Autodesk Fusion 360 part; units mm, degrees
(part 2 of 2)
sketch "Sketch26" plane through (0, 0, 45.5) normal (0, 0, 1) x (-1, 0, 0)
  line L0 (180, -249) -> (180, -94.7885)
  line L1 (180, -94.7885) -> (6, -94.7885)
  line L2 (6, -94.7885) -> (6, -109.4985)
  line L3 (6, -109.4985) -> (-58, -109.4985)
  line L4 (-58, -109.4985) -> (-58, -249)
  line L5 (-58, -249) -> (180, -249)
  circle A0 centre (58, -179.8487) radius 2.75
  circle A1 centre (58, -204.6724) radius 2.75
  circle A2 centre (58, -154.7263) radius 2.75
  circle A3 centre (58, -230.0227) radius 2.75
  circle A4 centre (58, -129.8013) radius 2.75
  line L6 (170, -234) -> (70, -234)
  line L7 (70, -229) -> (170, -229)
  arc A5 (170, -234) -> (170, -229) centre (170, -231.5) ccw
  arc A6 (70, -229) -> (70, -234) centre (70, -231.5) ccw
  line L8 (70, -219.3846) -> (170, -219.3846)
  line L9 (170, -224.3846) -> (70, -224.3846)
  arc A7 (170, -224.3846) -> (170, -219.3846) centre (170, -221.8846) ccw
  arc A8 (70, -219.3846) -> (70, -224.3846) centre (70, -221.8846) ccw
  line L10 (70, -209.7692) -> (170, -209.7692)
  line L11 (170, -214.7692) -> (70, -214.7692)
  arc A9 (170, -214.7692) -> (170, -209.7692) centre (170, -212.2692) ccw
  arc A10 (70, -209.7692) -> (70, -214.7692) centre (70, -212.2692) ccw
  line L12 (70, -200.1538) -> (170, -200.1538)
  line L13 (170, -205.1538) -> (70, -205.1538)
  arc A11 (170, -205.1538) -> (170, -200.1538) centre (170, -202.6538) ccw
  arc A12 (70, -200.1538) -> (70, -205.1538) centre (70, -202.6538) ccw
  line L14 (70, -180.9231) -> (170, -180.9231)
  line L15 (170, -185.9231) -> (70, -185.9231)
  arc A13 (170, -185.9231) -> (170, -180.9231) centre (170, -183.4231) ccw
  arc A14 (70, -180.9231) -> (70, -185.9231) centre (70, -183.4231) ccw
  line L16 (70, -152.0769) -> (170, -152.0769)
  line L17 (170, -157.0769) -> (70, -157.0769)
  arc A15 (170, -157.0769) -> (170, -152.0769) centre (170, -154.5769) ccw
  arc A16 (70, -152.0769) -> (70, -157.0769) centre (70, -154.5769) ccw
  line L18 (70, -123.2308) -> (170, -123.2308)
  line L19 (170, -128.2308) -> (70, -128.2308)
  arc A17 (170, -128.2308) -> (170, -123.2308) centre (170, -125.7308) ccw
  arc A18 (70, -123.2308) -> (70, -128.2308) centre (70, -125.7308) ccw
  line L20 (70, -104) -> (170, -104)
  line L21 (170, -109) -> (70, -109)
  arc A19 (170, -109) -> (170, -104) centre (170, -106.5) ccw
  arc A20 (70, -104) -> (70, -109) centre (70, -106.5) ccw
  dimension "d193" = 5
  dimension "d194" = 5
  dimension "d197" = 0
  dimension "d198" = 125
  constraint horizontal L6
  constraint horizontal L7
  measures "d193" diameter of A6
  measures "d194" diameter of A5
extrude "Extrude39" cut sketch "Sketch26" against normal blind 15 contours L6 L7 A5 A6 | L8 L9 A7 A8 | L10 L11 A9 A10 | L12 L13 A11 A12 | L14 L15 A13 A14 | L16 L17 A15 A16 | L18 L19 A17 A18 | L20 L21 A19 A20 bodies 8
sketch "Sketch27" plane through (0, 69, 0) normal (0, 1, 0) x (-1, 0, 0)
  line L0 (-29.7143, 10) -> (-29.7143, 35)
  arc A0 (-24.7143, 35) -> (-29.7143, 35) centre (-27.2143, 35) ccw
  line L1 (-24.7143, 35) -> (-24.7143, 10)
  arc A1 (-29.7143, 10) -> (-24.7143, 10) centre (-27.2143, 10) ccw
  line L2 (8.8571, 10) -> (8.8571, 35)
  arc A2 (13.8571, 35) -> (8.8571, 35) centre (11.3571, 35) ccw
  line L3 (13.8571, 35) -> (13.8571, 10)
  arc A3 (8.8571, 10) -> (13.8571, 10) centre (11.3571, 10) ccw
  line L4 (66.7143, 10) -> (66.7143, 35)
  arc A4 (71.7143, 35) -> (66.7143, 35) centre (69.2143, 35) ccw
  line L5 (71.7143, 35) -> (71.7143, 10)
  arc A5 (66.7143, 10) -> (71.7143, 10) centre (69.2143, 10) ccw
  line L6 (76.3571, 10) -> (76.3571, 35)
  arc A6 (81.3571, 35) -> (76.3571, 35) centre (78.8571, 35) ccw
  line L7 (81.3571, 35) -> (81.3571, 10)
  arc A7 (76.3571, 10) -> (81.3571, 10) centre (78.8571, 10) ccw
  line L8 (18.5, 10) -> (18.5, 35)
  arc A8 (23.5, 35) -> (18.5, 35) centre (21, 35) ccw
  line L9 (23.5, 35) -> (23.5, 10)
  arc A9 (18.5, 10) -> (23.5, 10) centre (21, 10) ccw
  line L10 (-20.0714, 10) -> (-20.0714, 35)
  arc A10 (-15.0714, 35) -> (-20.0714, 35) centre (-17.5714, 35) ccw
  line L11 (-15.0714, 35) -> (-15.0714, 10)
  arc A11 (-20.0714, 10) -> (-15.0714, 10) centre (-17.5714, 10) ccw
  line L12 (-39.3571, 10) -> (-39.3571, 35)
  arc A12 (-34.3571, 35) -> (-39.3571, 35) centre (-36.8571, 35) ccw
  line L13 (-34.3571, 35) -> (-34.3571, 10)
  arc A13 (-39.3571, 10) -> (-34.3571, 10) centre (-36.8571, 10) ccw
  line L14 (-0.7857, 10) -> (-0.7857, 35)
  arc A14 (4.2143, 35) -> (-0.7857, 35) centre (1.7143, 35) ccw
  line L15 (4.2143, 35) -> (4.2143, 10)
  arc A15 (-0.7857, 10) -> (4.2143, 10) centre (1.7143, 10) ccw
  line L16 (57.0714, 10) -> (57.0714, 35)
  arc A16 (62.0714, 35) -> (57.0714, 35) centre (59.5714, 35) ccw
  line L17 (62.0714, 35) -> (62.0714, 10)
  arc A17 (57.0714, 10) -> (62.0714, 10) centre (59.5714, 10) ccw
  line L18 (86, 10) -> (86, 35)
  arc A18 (91, 35) -> (86, 35) centre (88.5, 35) ccw
  line L19 (91, 35) -> (91, 10)
  arc A19 (86, 10) -> (91, 10) centre (88.5, 10) ccw
  line L20 (47.4286, 10) -> (47.4286, 35)
  arc A20 (52.4286, 35) -> (47.4286, 35) centre (49.9286, 35) ccw
  line L21 (52.4286, 35) -> (52.4286, 10)
  arc A21 (47.4286, 10) -> (52.4286, 10) centre (49.9286, 10) ccw
  line L22 (-10.4286, 10) -> (-10.4286, 35)
  arc A22 (-5.4286, 35) -> (-10.4286, 35) centre (-7.9286, 35) ccw
  line L23 (-5.4286, 35) -> (-5.4286, 10)
  arc A23 (-10.4286, 10) -> (-5.4286, 10) centre (-7.9286, 10) ccw
  line L24 (-49, 10) -> (-49, 35)
  arc A24 (-44, 35) -> (-49, 35) centre (-46.5, 35) ccw
  line L25 (-44, 35) -> (-44, 10)
  arc A25 (-49, 10) -> (-44, 10) centre (-46.5, 10) ccw
  line L26 (180, 3) -> (-58, 3)
  line L27 (180, 3) -> (180, 61)
  line L28 (180, 61) -> (-58, 61)
  line L29 (-58, 61) -> (-58, 3)
  circle A26 centre (34, 14) radius 7
  line L30 (100, 35) -> (100, 10)
  line L31 (95, 10) -> (95, 35)
  arc A27 (100, 35) -> (95, 35) centre (97.5, 35) ccw
  arc A28 (95, 10) -> (100, 10) centre (97.5, 10) ccw
  line L32 (109.7143, 35) -> (109.7143, 10)
  line L33 (104.7143, 10) -> (104.7143, 35)
  arc A29 (109.7143, 35) -> (104.7143, 35) centre (107.2143, 35) ccw
  arc A30 (104.7143, 10) -> (109.7143, 10) centre (107.2143, 10) ccw
  line L34 (119.4286, 35) -> (119.4286, 10)
  line L35 (114.4286, 10) -> (114.4286, 35)
  arc A31 (119.4286, 35) -> (114.4286, 35) centre (116.9286, 35) ccw
  arc A32 (114.4286, 10) -> (119.4286, 10) centre (116.9286, 10) ccw
  line L36 (129.1429, 35) -> (129.1429, 10)
  line L37 (124.1429, 10) -> (124.1429, 35)
  arc A33 (129.1429, 35) -> (124.1429, 35) centre (126.6429, 35) ccw
  arc A34 (124.1429, 10) -> (129.1429, 10) centre (126.6429, 10) ccw
  line L38 (138.8571, 35) -> (138.8571, 10)
  line L39 (133.8571, 10) -> (133.8571, 35)
  arc A35 (138.8571, 35) -> (133.8571, 35) centre (136.3571, 35) ccw
  arc A36 (133.8571, 10) -> (138.8571, 10) centre (136.3571, 10) ccw
  line L40 (148.5714, 35) -> (148.5714, 10)
  line L41 (143.5714, 10) -> (143.5714, 35)
  arc A37 (148.5714, 35) -> (143.5714, 35) centre (146.0714, 35) ccw
  arc A38 (143.5714, 10) -> (148.5714, 10) centre (146.0714, 10) ccw
  line L42 (158.2857, 35) -> (158.2857, 10)
  line L43 (153.2857, 10) -> (153.2857, 35)
  arc A39 (158.2857, 35) -> (153.2857, 35) centre (155.7857, 35) ccw
  arc A40 (153.2857, 10) -> (158.2857, 10) centre (155.7857, 10) ccw
  line L44 (168, 35) -> (168, 10)
  line L45 (163, 10) -> (163, 35)
  arc A41 (168, 35) -> (163, 35) centre (165.5, 35) ccw
  arc A42 (163, 10) -> (168, 10) centre (165.5, 10) ccw
  dimension "d201" = 5
  dimension "d202" = 5
  dimension "d205" = 68
  dimension "d206" = 0
  constraint vertical L30
  constraint vertical L31
  measures "d201" diameter of A27
  measures "d202" diameter of A28
sketch "Sketch28" plane through (0, 69, 0) normal (0, 1, 0) x (-1, 0, 0)
extrude "Extrude40" cut sketch "Sketch27" against normal blind 10 contours L30 L31 A27 A28 | L32 L33 A29 A30 | L34 L35 A31 A32 | L36 L37 A33 A34 | L38 L39 A35 A36 | L40 L41 A37 A38 | L42 L43 A39 A40 | L44 L45 A41 A42 bodies 2
fillet "Fillet16" radius 2.5 20 edges at (-95, -75.9913, 57) (-103, -75.9913, 57) (-111, -75.9913, 57) (-119, -75.9913, 57) (-127, -75.9913, 57) (-135, -76, 57) (-143, -76, 57) (-151, -76, 57) (-159, -76, 57) (-167, -75.9913, 57) (-172, -75.9913, 57) (-164, -75.9913, 57) (-156, -76, 57) (-148, -76, 57) (-140, -76, 57) (-132, -75.9913, 57) (-124, -75.9913, 57) (-116, -75.9913, 57) (-108, -75.9913, 57) (-100, -75.9913, 57) on bodies 2
extrude "Extrude41" cut sketch "Sketch23" against normal blind 235 bodies 2
sketch "Sketch29" plane through (0, -79, 0) normal (0, -1, 0) x (1, 0, 0)
  line L0 (-95, 54.5) -> (-95, 10)
  arc A0 (-100, 10) -> (-95, 10) centre (-97.5, 10) ccw
  line L1 (-100, 10) -> (-100, 54.5)
  arc A1 (-97.5, 57) -> (-100, 54.5) centre (-97.5, 54.5) ccw
  arc A2 (-95, 54.5) -> (-97.5, 57) centre (-97.5, 54.5) ccw
  line L2 (-8.0005, 61) -> (-180, 61)
  line L3 (-180, 61) -> (-180, 3)
  line L4 (-8.0005, 3) -> (-180, 3)
  line L5 (-8.0005, 3) -> (-8.0005, 61)
  line L6 (-167, 54.5) -> (-167, 10)
  arc A3 (-172, 10) -> (-167, 10) centre (-169.5, 10) ccw
  line L7 (-172, 10) -> (-172, 54.5)
  arc A4 (-169.5, 57) -> (-172, 54.5) centre (-169.5, 54.5) ccw
  arc A5 (-167, 54.5) -> (-169.5, 57) centre (-169.5, 54.5) ccw
  line L8 (-159, 54.5) -> (-159, 10)
  arc A6 (-164, 10) -> (-159, 10) centre (-161.5, 10) ccw
  line L9 (-164, 10) -> (-164, 54.5)
  arc A7 (-161.5, 57) -> (-164, 54.5) centre (-161.5, 54.5) ccw
  arc A8 (-159, 54.5) -> (-161.5, 57) centre (-161.5, 54.5) ccw
  line L10 (-151, 54.5) -> (-151, 10)
  arc A9 (-156, 10) -> (-151, 10) centre (-153.5, 10) ccw
  line L11 (-156, 10) -> (-156, 54.5)
  arc A10 (-153.5, 57) -> (-156, 54.5) centre (-153.5, 54.5) ccw
  arc A11 (-151, 54.5) -> (-153.5, 57) centre (-153.5, 54.5) ccw
  line L12 (-143, 54.5) -> (-143, 10)
  arc A12 (-148, 10) -> (-143, 10) centre (-145.5, 10) ccw
  line L13 (-148, 10) -> (-148, 54.5)
  arc A13 (-145.5, 57) -> (-148, 54.5) centre (-145.5, 54.5) ccw
  arc A14 (-143, 54.5) -> (-145.5, 57) centre (-145.5, 54.5) ccw
  line L14 (-135, 54.5) -> (-135, 10)
  arc A15 (-140, 10) -> (-135, 10) centre (-137.5, 10) ccw
  line L15 (-140, 10) -> (-140, 54.5)
  arc A16 (-137.5, 57) -> (-140, 54.5) centre (-137.5, 54.5) ccw
  arc A17 (-135, 54.5) -> (-137.5, 57) centre (-137.5, 54.5) ccw
  line L16 (-127, 54.5) -> (-127, 10)
  arc A18 (-132, 10) -> (-127, 10) centre (-129.5, 10) ccw
  line L17 (-132, 10) -> (-132, 54.5)
  arc A19 (-129.5, 57) -> (-132, 54.5) centre (-129.5, 54.5) ccw
  arc A20 (-127, 54.5) -> (-129.5, 57) centre (-129.5, 54.5) ccw
  line L18 (-119, 54.5) -> (-119, 10)
  arc A21 (-124, 10) -> (-119, 10) centre (-121.5, 10) ccw
  line L19 (-124, 10) -> (-124, 54.5)
  arc A22 (-121.5, 57) -> (-124, 54.5) centre (-121.5, 54.5) ccw
  arc A23 (-119, 54.5) -> (-121.5, 57) centre (-121.5, 54.5) ccw
  line L20 (-111, 54.5) -> (-111, 10)
  arc A24 (-116, 10) -> (-111, 10) centre (-113.5, 10) ccw
  line L21 (-116, 10) -> (-116, 54.5)
  arc A25 (-113.5, 57) -> (-116, 54.5) centre (-113.5, 54.5) ccw
  arc A26 (-111, 54.5) -> (-113.5, 57) centre (-113.5, 54.5) ccw
  line L22 (-103, 54.5) -> (-103, 10)
  arc A27 (-108, 10) -> (-103, 10) centre (-105.5, 10) ccw
  line L23 (-108, 10) -> (-108, 54.5)
  arc A28 (-105.5, 57) -> (-108, 54.5) centre (-105.5, 54.5) ccw
  arc A29 (-103, 54.5) -> (-105.5, 57) centre (-105.5, 54.5) ccw
  line L24 (-158, 20) -> (-93.1453, 20)
  line L25 (-93.1453, 20) -> (-93.1453, 7.5)
  line L26 (-93.1453, 7.5) -> (-158, 7.5)
  line L27 (-158, 7.5) -> (-158, 20)
  line L28 (-164, 23) -> (-90, 23)
  line L29 (-90, 23) -> (-90, 6)
  line L30 (-90, 6) -> (-164, 6)
  line L31 (-164, 6) -> (-164, 23)
  constraint horizontal L24
  constraint vertical L25
  constraint horizontal L26
  constraint vertical L27
  constraint horizontal L28
  constraint vertical L29
  constraint horizontal L30
  constraint vertical L31
  constraint coincident L9 L28.start
extrude "Extrude42" cut sketch "Sketch29" against normal blind 10 contours L0 A0 L24 L25 L26 | A0 L1 L22 A27 L24 L26 | L20 A24 A27 L23 L24 L26 | L18 A21 A24 L21 L24 L26 | L16 A18 A21 L19 L24 L26 | L14 A15 A18 L17 L24 L26 | L12 A12 A15 L15 L24 L26 | A9 L11 L24 L26 L27 | L10 A9 A12 L13 L24 L26 bodies 2
extrude "Extrude43" add sketch "Sketch29" against normal blind 6 contours L0 L1 L24 L28 | L22 L23 L24 L28 | L20 L21 L24 L28 | L8 A6 L9 L28 L31 | L18 L19 L24 L28 | L10 L11 L24 L28 | L16 L17 L24 L28 | L12 L13 L24 L28 | L14 L15 L24 L28 bodies 2
fillet "Fillet17" radius 2.5 1 edges at (-127, -76, 23) on bodies 2
fillet "Fillet18" radius 2.5 9 edges at (-132, -76, 23) (-140, -76, 23) (-148, -76, 23) (-156, -76, 23) (-164, -76, 23) (-124, -76, 23) (-116, -76, 23) (-108, -76, 23) (-100, -76, 23) on bodies 2
fillet "Fillet19" radius 2.5 8 edges at (-95, -76, 23) (-103, -76, 23) (-111, -76, 23) (-119, -76, 23) (-135, -76, 23) (-143, -76, 23) (-151, -76, 23) (-159, -76, 23) on bodies 2
fillet "Fillet20" radius 3 2 edges at (-93.1453, -75.9913, 20) (-93.1453, -75.9913, 7.5) on bodies 2
extrude "Extrude44" cut 1 faces at (-158, -77, 11.6667) along direction (-1, 0, 0) blind 6 on bodies 2 bodies 2
fillet "Fillet21" radius 3 2 edges at (-164, -76, 20) (-164, -76, 7.5) on bodies 2
sketch "Sketch30" plane through (-0.0009, 63.0004, 0) normal (0.000014, -1, 0) x (1, 0.000014, 0)
  line L0 (-49.9991, 7.501) -> (-49.9991, 4)
  line L1 (-49.9991, 4) -> (52.0207, 4)
  line L2 (52.0207, 4) -> (52.0207, 58)
  line L3 (52.0207, 58) -> (-49.9991, 58)
  line L4 (-49.9991, 58) -> (-49.9991, 37.499)
  arc A0 (-47.4277, 35) -> (-49.9991, 37.499) centre (-49.9277, 35) ccw
  line L5 (-47.4277, 35) -> (-47.4277, 10)
  arc A1 (-49.9991, 7.501) -> (-47.4277, 10) centre (-49.9277, 10) ccw
  line L6 (49.0009, 35) -> (49.0009, 10)
  arc A2 (44.0009, 10) -> (49.0009, 10) centre (46.5009, 10) ccw
  line L7 (44.0009, 10) -> (44.0009, 35)
  arc A3 (49.0009, 35) -> (44.0009, 35) centre (46.5009, 35) ccw
  line L8 (10.4295, 35) -> (10.4295, 10)
  arc A4 (5.4295, 10) -> (10.4295, 10) centre (7.9295, 10) ccw
  line L9 (5.4295, 10) -> (5.4295, 35)
  arc A5 (10.4295, 35) -> (5.4295, 35) centre (7.9295, 35) ccw
  line L10 (0.7866, 35) -> (0.7866, 10)
  arc A6 (-4.2134, 10) -> (0.7866, 10) centre (-1.7134, 10) ccw
  line L11 (-4.2134, 10) -> (-4.2134, 35)
  arc A7 (0.7866, 35) -> (-4.2134, 35) centre (-1.7134, 35) ccw
  line L12 (39.358, 35) -> (39.358, 10)
  arc A8 (34.358, 10) -> (39.358, 10) centre (36.858, 10) ccw
  line L13 (34.358, 10) -> (34.358, 35)
  arc A9 (39.358, 35) -> (34.358, 35) centre (36.858, 35) ccw
  line L14 (20.0723, 35) -> (20.0723, 10)
  arc A10 (15.0723, 10) -> (20.0723, 10) centre (17.5723, 10) ccw
  line L15 (15.0723, 10) -> (15.0723, 35)
  arc A11 (20.0723, 35) -> (15.0723, 35) centre (17.5723, 35) ccw
  line L16 (-18.4991, 35) -> (-18.4991, 10)
  arc A12 (-23.4991, 10) -> (-18.4991, 10) centre (-20.9991, 10) ccw
  line L17 (-23.4991, 10) -> (-23.4991, 35)
  arc A13 (-18.4991, 35) -> (-23.4991, 35) centre (-20.9991, 35) ccw
  line L18 (-8.8563, 35) -> (-8.8563, 10)
  arc A14 (-13.8563, 10) -> (-8.8563, 10) centre (-11.3563, 10) ccw
  line L19 (-13.8563, 10) -> (-13.8563, 35)
  arc A15 (-8.8563, 35) -> (-13.8563, 35) centre (-11.3563, 35) ccw
  line L20 (29.7152, 35) -> (29.7152, 10)
  arc A16 (24.7152, 10) -> (29.7152, 10) centre (27.2152, 10) ccw
  line L21 (24.7152, 10) -> (24.7152, 35)
  arc A17 (29.7152, 35) -> (24.7152, 35) centre (27.2152, 35) ccw
  circle A18 centre (-33.9991, 14) radius 7
  circle A19 centre (30, 50) radius 3.25
  circle A20 centre (0, 50) radius 3.25
  circle A21 centre (-30, 50) radius 3.25
  circle A22 centre (-75, 50) radius 3.25
  circle A23 centre (-115, 50) radius 3.25
  circle A24 centre (-155, 50) radius 3.25
  dimension "d229" = 6.5
  dimension "d230" = 6.5
  dimension "d231" = 6.5
  dimension "d232" = 30
  dimension "d233" = 30
  dimension "d234" = 6.5
  dimension "d237" = -80
  dimension "d238" = 0
  measures "d229" diameter of A19
  measures "d230" diameter of A20
  measures "d231" diameter of A21
  measures "d232" distance of A19.centre A20.centre
  measures "d233" distance of A20.centre A21.centre
  measures "d234" diameter of A22
extrude "Extrude45" cut sketch "Sketch30" against normal blind 20 contours A19 | A20 | A21 | A22 | A23 | A24 bodies 2
